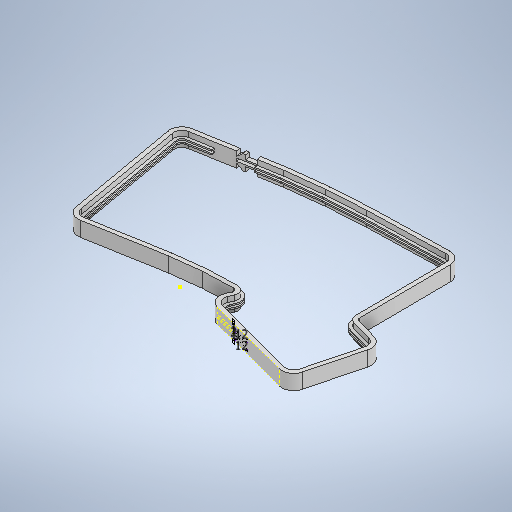
# Autodesk Inventor part: Case2.0_whole
Saved by Autodesk Inventor 2025 (Build 290162000, 162)
## iProperties
Created: 2024-07-14
Part Number: Case2.0_whole
Material: Generic
Document SubType Name: Modeling
Designer: ethan
Density: 1 g/cm^3
Appearance: Default
Author: ethan
Autodesk Inventor part; units mm, degrees
ref_plane "YZ Plane" through (0, 0, 0) normal (1, 0, 0) x (0, 1, 0)
ref_plane "XZ Plane" through (0, 0, 0) normal (0, 1, 0) x (-1, 0, 0)
sketch "Sketch1" plane through (0, 0, 0) normal (0, 1, 0) x (-1, 0, 0)
  line L0 (-82.0743, -49.0378) -> (-95.2699, 25.7981) construction
  line L1 (-91.2026, 31.5924) -> (-36.7795, 41.0576) construction
  line L2 (-36.5045, 41.0976) -> (-11.557, 44.02) construction
  line L3 (-11.2903, 44.0441) -> (14.1113, 45.648) construction
  line L4 (14.295, 45.6562) -> (66.1055, 47.0175) construction
  line L5 (71.2366, 42.0628) -> (71.7707, -19.1365) construction
  line L6 (75.3629, -23.8906) -> (89.6926, -28.0947) construction
  line L7 (93.1258, -34.1444) -> (84.0794, -69.1243) construction
  line L8 (77.9595, -72.706) -> (21.637, -57.8008) construction
  line L9 (18.302, -51.0413) -> (19.5764, -47.9879) construction
  line L10 (14.7916, -41.0649) -> (-5.2075, -41.7475) construction
  line L11 (-5.6408, -41.7811) -> (-26.0301, -44.2616) construction
  line L12 (-26.2924, -44.3006) -> (-76.2841, -53.0939) construction
  arc A0 (-91.2026, 31.5924) -> (-95.2699, 25.7981) centre (-90.3459, 26.6664) ccw construction
  arc A1 (-36.5045, 41.0976) -> (-36.7795, 41.0576) centre (-35.9227, 36.1315) ccw construction
  arc A2 (-11.2903, 44.0441) -> (-11.557, 44.02) centre (-10.9752, 39.054) ccw construction
  arc A3 (14.295, 45.6562) -> (14.1113, 45.648) centre (14.4264, 40.6579) ccw construction
  arc A4 (71.2366, 42.0628) -> (66.1055, 47.0175) centre (66.2368, 42.0192) ccw construction
  arc A5 (71.7707, -19.1365) -> (75.3629, -23.8906) centre (76.7705, -19.0928) ccw construction
  arc A6 (93.1258, -34.1444) -> (89.6926, -28.0947) centre (88.285, -32.8925) ccw construction
  arc A7 (77.9595, -72.706) -> (84.0794, -69.1243) centre (79.2386, -67.8724) ccw construction
  arc A8 (18.302, -51.0413) -> (21.637, -57.8008) centre (22.9162, -52.9672) ccw construction
  arc A9 (19.5764, -47.9879) -> (14.7916, -41.0649) centre (14.9621, -46.062) ccw construction
  arc A10 (-5.2075, -41.7475) -> (-5.6408, -41.7811) centre (-5.037, -46.7446) ccw construction
  arc A11 (-26.0301, -44.2616) -> (-26.2924, -44.3006) centre (-25.4262, -49.225) ccw construction
  arc A12 (-82.0743, -49.0378) -> (-76.2841, -53.0939) centre (-77.1503, -48.1695) ccw construction
  arc A13 (-91.2369, 31.7895) -> (-95.4669, 25.7634) centre (-90.3459, 26.6664) ccw
  line L13 (-91.2369, 31.7895) -> (-36.8137, 41.2546)
  arc A14 (-36.5277, 41.2962) -> (-36.8137, 41.2546) centre (-35.9227, 36.1315) ccw
  line L14 (-36.5277, 41.2962) -> (-11.5803, 44.2187)
  line L15 (-11.3029, 44.2437) -> (14.0987, 45.8476)
  arc A15 (-11.3029, 44.2437) -> (-11.5803, 44.2187) centre (-10.9752, 39.054) ccw
  arc A16 (14.2898, 45.8561) -> (14.0987, 45.8476) centre (14.4264, 40.6579) ccw
  line L16 (14.2898, 45.8561) -> (66.1002, 47.2174)
  arc A17 (71.4366, 42.0646) -> (66.1002, 47.2174) centre (66.2368, 42.0192) ccw
  line L17 (71.4366, 42.0646) -> (71.9707, -19.1347)
  arc A18 (71.9707, -19.1347) -> (75.4192, -23.6987) centre (76.7705, -19.0928) ccw
  line L18 (75.4192, -23.6987) -> (89.7489, -27.9028)
  arc A19 (93.3194, -34.1945) -> (89.7489, -27.9028) centre (88.285, -32.8925) ccw
  line L19 (93.3194, -34.1945) -> (84.273, -69.1743)
  arc A20 (77.9083, -72.8993) -> (84.273, -69.1743) centre (79.2386, -67.8724) ccw
  line L20 (77.9083, -72.8993) -> (21.5859, -57.9941)
  arc A21 (18.1174, -50.9643) -> (21.5859, -57.9941) centre (22.9162, -52.9672) ccw
  line L21 (18.1174, -50.9643) -> (19.3918, -47.9108)
  arc A22 (19.3918, -47.9108) -> (14.7984, -41.2648) centre (14.9621, -46.062) ccw
  line L22 (14.7984, -41.2648) -> (-5.2007, -41.9473)
  arc A23 (-5.2007, -41.9473) -> (-5.6167, -41.9797) centre (-5.037, -46.7446) ccw
  line L23 (-5.6167, -41.9797) -> (-26.0059, -44.4601)
  arc A24 (-26.0059, -44.4601) -> (-26.2578, -44.4975) centre (-25.4262, -49.225) ccw
  line L24 (-26.2578, -44.4975) -> (-76.2494, -53.2909)
  arc A25 (-82.2713, -49.0725) -> (-76.2494, -53.2909) centre (-77.1503, -48.1695) ccw
  line L25 (-82.2713, -49.0725) -> (-95.4669, 25.7634)
  arc A26 (-91.7166, 34.5481) -> (-98.2243, 25.2772) centre (-90.3459, 26.6664) ccw
  line L26 (-91.7166, 34.5481) -> (-37.2935, 44.0132)
  line L27 (-36.8535, 44.0772) -> (-11.906, 46.9997)
  arc A27 (-36.8535, 44.0772) -> (-37.2935, 44.0132) centre (-35.9227, 36.1315) ccw
  arc A28 (-11.4794, 47.0381) -> (-11.906, 46.9997) centre (-10.9752, 39.054) ccw
  line L28 (-11.4794, 47.0381) -> (13.9222, 48.642)
  arc A29 (14.2162, 48.6551) -> (13.9222, 48.642) centre (14.4264, 40.6579) ccw
  line L29 (14.2162, 48.6551) -> (66.0267, 50.0164)
  arc A30 (74.2365, 42.089) -> (66.0267, 50.0164) centre (66.2368, 42.0192) ccw
  line L30 (74.2365, 42.089) -> (74.7706, -19.1103)
  arc A31 (74.7706, -19.1103) -> (76.2074, -21.0119) centre (76.7705, -19.0928) ccw
  line L31 (76.2074, -21.0119) -> (90.5372, -25.2161)
  arc A32 (96.0302, -34.8956) -> (90.5372, -25.2161) centre (88.285, -32.8925) ccw
  line L32 (96.0302, -34.8956) -> (86.9838, -69.8754)
  arc A33 (77.192, -75.6061) -> (86.9838, -69.8754) centre (79.2386, -67.8724) ccw
  line L33 (77.192, -75.6061) -> (20.8695, -60.7009)
  arc A34 (15.5334, -49.8859) -> (20.8695, -60.7009) centre (22.9162, -52.9672) ccw
  arc A35 (16.8078, -46.8324) -> (14.8939, -44.0632) centre (14.9621, -46.062) ccw
  line L34 (15.5334, -49.8859) -> (16.8078, -46.8324)
  line L35 (14.8939, -44.0632) -> (-5.1052, -44.7457)
  arc A36 (-5.1052, -44.7457) -> (-5.2785, -44.7592) centre (-5.037, -46.7446) ccw
  line L36 (-5.2785, -44.7592) -> (-25.6678, -47.2396)
  arc A37 (-25.6678, -47.2396) -> (-25.7727, -47.2552) centre (-25.4262, -49.225) ccw
  line L37 (-25.7727, -47.2552) -> (-75.7644, -56.0486)
  line L38 (-85.0287, -49.5587) -> (-98.2243, 25.2772)
  arc A38 (-85.0287, -49.5587) -> (-75.7644, -56.0486) centre (-77.1503, -48.1695) ccw
  point P0 (-26.1615, -44.2793)
  point P1 (-5.4246, -41.7596)
  point P2 (14.2031, 45.6529)
  point P3 (-25.7727, -47.2552)
  point P4 (-25.6678, -47.2396)
  point P5 (-5.2785, -44.7592)
  point P6 (-5.1052, -44.7457)
  point P7 (14.8939, -44.0632)
  point P8 (16.8078, -46.8324)
  point P9 (76.2074, -21.0119)
  point P10 (74.7706, -19.1103)
  point P11 (74.2365, 42.089)
  point P12 (-11.5803, 44.2187)
  point P13 (71.9707, -19.1347)
  point P14 (75.4192, -23.6987)
  point P15 (-5.2007, -41.9473)
  point P16 (-5.6167, -41.9797)
  point P17 (-26.2578, -44.4975)
  point P18 (-95.4669, 25.7634)
  dimension "d8" = 0.2
  dimension "d9" = 0.2
  dimension "d10" = 0.2
  dimension "d11" = 0.2
  dimension "d12" = 0.2
  dimension "d13" = 0.2
  dimension "d14" = 0.2
  dimension "d15" = 0.2
  dimension "d16" = 0.2
  dimension "d17" = 0.2
  dimension "d18" = 0.2
  dimension "d19" = 0.2
  dimension "d20" = 0.2
  dimension "d21" = 0.2
  dimension "d22" = 0.2
  dimension "d23" = 0.2
  dimension "d24" = 0.2
  dimension "d25" = 0.2
  dimension "d26" = 0.2
  dimension "d27" = 0.2
  dimension "d28" = 0.2
  dimension "d29" = 0.2
  dimension "d30" = 0.2
  dimension "d31" = 0.2
  dimension "d32" = 0.2
  dimension "d33" = 0.2
  dimension "d34" = 2.8
  dimension "d35" = 2.8
  dimension "d36" = 2.8
  dimension "d37" = 2.8
  dimension "d38" = 2.8
  dimension "d39" = 2.8
  dimension "d40" = 2.8
  dimension "d41" = 2.8
  dimension "d42" = 2.8
  dimension "d43" = 2.8
  dimension "d44" = 2.8
  dimension "d45" = 2.8
  dimension "d46" = 2.8
  dimension "d47" = 2.8
  dimension "d48" = 2.8
  dimension "d49" = 2.8
  dimension "d50" = 2.8
  dimension "d51" = 2.8
  dimension "d52" = 2.8
  dimension "d53" = 2.8
  dimension "d54" = 2.8
  dimension "d55" = 2.8
  dimension "d56" = 2.8
  dimension "d57" = 2.8
  dimension "d58" = 2.8
  dimension "d59" = 2.8
  constraints: 81 point on circle, 78 end point, 39 centre point, 26 parallel, 33 other
  measures "d8" radial gap between concentric circles of A0 A13
  measures "d9" distance between parallel lines of L1 L13
  measures "d10" radial gap between concentric circles of A1 A14
  measures "d11" distance between parallel lines of L2 L14
  measures "d12" distance between parallel lines of L3 L15
  measures "d13" radial gap between concentric circles of A2 A15
  measures "d14" radial gap between concentric circles of A3 A16
  measures "d15" distance between parallel lines of L4 L16
  measures "d16" radial gap between concentric circles of A4 A17
  measures "d17" distance between parallel lines of L5 L17
  measures "d18" radial gap between concentric circles of A5 A18
  measures "d19" distance between parallel lines of L6 L18
  measures "d20" radial gap between concentric circles of A6 A19
  measures "d21" distance between parallel lines of L7 L19
  measures "d22" radial gap between concentric circles of A7 A20
  measures "d23" distance between parallel lines of L8 L20
  measures "d24" radial gap between concentric circles of A8 A21
  measures "d25" distance between parallel lines of L9 L21
  measures "d26" radial gap between concentric circles of A9 A22
  measures "d27" distance between parallel lines of L10 L22
  measures "d28" radial gap between concentric circles of A10 A23
  measures "d29" distance between parallel lines of L11 L23
  measures "d30" radial gap between concentric circles of A11 A24
  measures "d31" distance between parallel lines of L12 L24
  measures "d32" radial gap between concentric circles of A12 A25
  measures "d33" distance between parallel lines of L0 L25
  measures "d34" radial gap between concentric circles of A13 A26
  measures "d35" distance between parallel lines of L13 L26
  measures "d36" distance between parallel lines of L14 L27
  measures "d37" radial gap between concentric circles of A14 A27
  measures "d38" radial gap between concentric circles of A15 A28
  measures "d39" distance between parallel lines of L15 L28
  measures "d40" radial gap between concentric circles of A16 A29
  measures "d41" distance between parallel lines of L16 L29
  measures "d42" radial gap between concentric circles of A17 A30
  measures "d43" distance between parallel lines of L17 L30
  measures "d44" radial gap between concentric circles of A18 A31
  measures "d45" distance between parallel lines of L18 L31
  measures "d46" radial gap between concentric circles of A19 A32
  measures "d47" distance between parallel lines of L19 L32
  measures "d48" radial gap between concentric circles of A20 A33
  measures "d49" distance between parallel lines of L20 L33
  measures "d50" radial gap between concentric circles of A21 A34
  measures "d51" radial gap between concentric circles of A22 A35
  measures "d52" distance between parallel lines of L21 L34
  measures "d53" distance between parallel lines of L22 L35
  measures "d54" radial gap between concentric circles of A23 A36
  measures "d55" distance between parallel lines of L23 L36
  measures "d56" radial gap between concentric circles of A24 A37
  measures "d57" distance between parallel lines of L24 L37
  measures "d58" distance between parallel lines of L25 L38
  measures "d59" radial gap between concentric circles of A25 A38
extrude "Body" add sketch "Sketch1" along normal blind 10
ref_plane "Midplane" through (0, 5, 0) normal (0, 1, 0) x (1, 0, 0)
sketch "Sketch2" plane through (0, 5, 0) normal (0, 1, 0) x (1, 0, 0)
  line L0 (37.2935, -44.0132) -> (91.7166, -34.5481) projected
  arc A0 (91.7166, -34.5481) -> (98.2243, -25.2772) centre (90.3459, -26.6664) ccw projected
  line L1 (98.2243, -25.2772) -> (85.0287, 49.5587) projected
  arc A1 (85.0287, 49.5587) -> (75.7644, 56.0486) centre (77.1503, 48.1695) ccw projected
  line L2 (75.7644, 56.0486) -> (25.7727, 47.2552) projected
  arc A2 (25.6678, 47.2396) -> (25.7727, 47.2552) centre (25.4262, 49.225) ccw projected
  line L3 (25.6678, 47.2396) -> (5.2785, 44.7592) projected
  arc A3 (5.1052, 44.7457) -> (5.2785, 44.7592) centre (5.037, 46.7446) ccw projected
  line L4 (5.1052, 44.7457) -> (-14.8939, 44.0632) projected
  arc A4 (-16.8078, 46.8324) -> (-14.8939, 44.0632) centre (-14.9621, 46.062) ccw projected
  line L5 (-16.8078, 46.8324) -> (-15.5334, 49.8859) projected
  arc A5 (-15.5334, 49.8859) -> (-20.8695, 60.7009) centre (-22.9162, 52.9672) ccw projected
  line L6 (-20.8695, 60.7009) -> (-77.192, 75.6061) projected
  arc A6 (-77.192, 75.6061) -> (-86.9838, 69.8754) centre (-79.2386, 67.8724) ccw projected
  line L7 (-86.9838, 69.8754) -> (-96.0302, 34.8956) projected
  arc A7 (-96.0302, 34.8956) -> (-90.5372, 25.2161) centre (-88.285, 32.8925) ccw projected
  line L8 (-90.5372, 25.2161) -> (-76.2074, 21.0119) projected
  arc A8 (-74.7706, 19.1103) -> (-76.2074, 21.0119) centre (-76.7705, 19.0928) ccw projected
  line L9 (-74.7706, 19.1103) -> (-74.2365, -42.089) projected
  arc A9 (-74.2365, -42.089) -> (-66.0267, -50.0164) centre (-66.2368, -42.0192) ccw projected
  line L10 (-66.0267, -50.0164) -> (-14.2162, -48.6551) projected
  arc A10 (-14.2162, -48.6551) -> (-13.9222, -48.642) centre (-14.4264, -40.6579) ccw projected
  line L11 (-13.9222, -48.642) -> (11.4794, -47.0381) projected
  arc A11 (11.4794, -47.0381) -> (11.906, -46.9997) centre (10.9752, -39.054) ccw projected
  line L12 (11.906, -46.9997) -> (36.8535, -44.0772) projected
  arc A12 (36.8535, -44.0772) -> (37.2935, -44.0132) centre (35.9227, -36.1315) ccw projected
  line L13 (36.5277, -41.2962) -> (11.5803, -44.2187) projected
  arc A13 (11.3029, -44.2437) -> (11.5803, -44.2187) centre (10.9752, -39.054) ccw projected
  line L14 (11.3029, -44.2437) -> (-14.0987, -45.8476) projected
  arc A14 (-14.2898, -45.8561) -> (-14.0987, -45.8476) centre (-14.4264, -40.6579) ccw projected
  line L15 (-14.2898, -45.8561) -> (-66.1002, -47.2174) projected
  arc A15 (-71.4366, -42.0646) -> (-66.1002, -47.2174) centre (-66.2368, -42.0192) ccw projected
  line L16 (-71.4366, -42.0646) -> (-71.9707, 19.1347) projected
  arc A16 (-71.9707, 19.1347) -> (-75.4192, 23.6987) centre (-76.7705, 19.0928) ccw projected
  line L17 (-75.4192, 23.6987) -> (-89.7489, 27.9028) projected
  arc A17 (-93.3194, 34.1945) -> (-89.7489, 27.9028) centre (-88.285, 32.8925) ccw projected
  line L18 (-93.3194, 34.1945) -> (-84.273, 69.1743) projected
  arc A18 (-77.9083, 72.8993) -> (-84.273, 69.1743) centre (-79.2386, 67.8724) ccw projected
  line L19 (-77.9083, 72.8993) -> (-21.5859, 57.9941) projected
  arc A19 (-18.1174, 50.9643) -> (-21.5859, 57.9941) centre (-22.9162, 52.9672) ccw projected
  line L20 (-18.1174, 50.9643) -> (-19.3918, 47.9108) projected
  arc A20 (-19.3918, 47.9108) -> (-14.7984, 41.2648) centre (-14.9621, 46.062) ccw projected
  line L21 (-14.7984, 41.2648) -> (5.2007, 41.9473) projected
  arc A21 (5.2007, 41.9473) -> (5.6167, 41.9797) centre (5.037, 46.7446) ccw projected
  line L22 (5.6167, 41.9797) -> (26.0059, 44.4601) projected
  arc A22 (26.0059, 44.4601) -> (26.2578, 44.4975) centre (25.4262, 49.225) ccw projected
  line L23 (26.2578, 44.4975) -> (76.2494, 53.2909) projected
  arc A23 (82.2713, 49.0725) -> (76.2494, 53.2909) centre (77.1503, 48.1695) ccw projected
  line L24 (82.2713, 49.0725) -> (95.4669, -25.7634) projected
  arc A24 (91.2369, -31.7895) -> (95.4669, -25.7634) centre (90.3459, -26.6664) ccw projected
  line L25 (91.2369, -31.7895) -> (36.8137, -41.2546) projected
  arc A25 (36.5277, -41.2962) -> (36.8137, -41.2546) centre (35.9227, -36.1315) ccw projected
  line L26 (-82.3367, 68.6736) -> (-91.3831, 33.6937)
  arc A26 (-91.3831, 33.6937) -> (-89.1859, 29.8219) centre (-88.285, 32.8925) ccw
  line L27 (-89.1859, 29.8219) -> (-74.8562, 25.6178)
  arc A27 (-69.9707, 19.1522) -> (-74.8562, 25.6178) centre (-76.7705, 19.0928) ccw
  line L28 (-69.9707, 19.1522) -> (-69.4367, -42.0471)
  arc A28 (-69.4367, -42.0471) -> (-66.1527, -45.2181) centre (-66.2368, -42.0192) ccw
  line L29 (-66.1527, -45.2181) -> (-14.3423, -43.8568)
  arc A29 (-14.3423, -43.8568) -> (-14.2247, -43.8515) centre (-14.4264, -40.6579) ccw
  line L30 (-14.2247, -43.8515) -> (11.1769, -42.2476)
  arc A30 (11.1769, -42.2476) -> (11.3476, -42.2323) centre (10.9752, -39.054) ccw
  line L31 (11.3476, -42.2323) -> (36.295, -39.3098)
  arc A31 (36.295, -39.3098) -> (36.471, -39.2842) centre (35.9227, -36.1315) ccw
  line L32 (36.471, -39.2842) -> (90.8942, -29.819)
  arc A32 (90.8942, -29.819) -> (93.4972, -26.1107) centre (90.3459, -26.6664) ccw
  line L33 (93.4972, -26.1107) -> (80.3017, 48.7252)
  arc A33 (80.3017, 48.7252) -> (76.5959, 51.3212) centre (77.1503, 48.1695) ccw
  line L34 (76.5959, 51.3212) -> (26.6043, 42.5278)
  arc A34 (26.2474, 42.4747) -> (26.6043, 42.5278) centre (25.4262, 49.225) ccw
  line L35 (26.2474, 42.4747) -> (5.8582, 39.9943)
  arc A35 (5.2689, 39.9485) -> (5.8582, 39.9943) centre (5.037, 46.7446) ccw
  line L36 (5.2689, 39.9485) -> (-14.7302, 39.266)
  arc A36 (-21.2375, 48.6811) -> (-14.7302, 39.266) centre (-14.9621, 46.062) ccw
  line L37 (-21.2375, 48.6811) -> (-19.9631, 51.7346)
  arc A37 (-19.9631, 51.7346) -> (-22.0975, 56.0607) centre (-22.9162, 52.9672) ccw
  line L38 (-22.0975, 56.0607) -> (-78.42, 70.9659)
  arc A38 (-78.42, 70.9659) -> (-82.3367, 68.6736) centre (-79.2386, 67.8724) ccw
  line L39 (63.6826, -34.5516) -> (64.0253, -36.522)
  line L40 (75.9977, -32.4098) -> (76.3404, -34.3802)
  line L41 (76.3404, -34.3802) -> (51.7102, -38.6639)
  line L42 (51.7102, -38.6639) -> (51.3675, -36.6934)
  line L43 (51.3675, -36.6934) -> (75.9977, -32.4098)
  line L44 (75.9977, -32.4098) -> (51.7102, -38.6639) construction
  line L45 (76.3404, -34.3802) -> (51.3675, -36.6934) construction
  line L46 (-50.2588, 63.5133) -> (-49.7471, 65.4467)
  line L47 (-61.8311, 68.6446) -> (-62.3428, 66.7112)
  line L48 (-62.3428, 66.7112) -> (-38.1747, 60.3154)
  line L49 (-38.1747, 60.3154) -> (-37.6631, 62.2488)
  line L50 (-37.6631, 62.2488) -> (-61.8311, 68.6446)
  line L51 (-61.8311, 68.6446) -> (-38.1747, 60.3154) construction
  line L52 (-62.3428, 66.7112) -> (-37.6631, 62.2488) construction
  point P0 (0, 0)
  point P1 (63.8539, -35.5368)
  point P2 (51.7102, -38.6639)
  point P3 (51.3675, -36.6934)
  point P4 (75.9977, -32.4098)
  point P5 (76.3404, -34.3802)
  point P6 (-50.0029, 64.48)
  point P7 (-61.8311, 68.6446)
  point P8 (-38.1747, 60.3154)
  dimension "d62" = 2
  dimension "d67" = 25
  dimension "d68" = 25
  constraints: 54 end point, 26 point on circle, 13 centre point, 10 midpoint, 5 parallel, 3 perpendicular, 25 other
  measures "d62" distance between parallel lines of L18 L26
  measures "d67" distance of L40.end L41.end
  measures "d68" distance of L48.end L47.end
extrude "Groove-Outer" add sketch "Sketch2" along normal mid plane 3 contours L13 A13 L14 A14 L15 A15 L16 A16 L17 A17 L18 A18 L19 L47 L38 A38 L26 A26 L27 A27 L28 A28 L29 A29 L30 A30 L31 A31 L32 L42 L25 A25 | L40 L32 A32 L33 A33 L34 A34 L35 A35 L36 A36 L37 A37 L38 L49 L19 A19 L20 A20 L21 A21 L22 A22 L23 A23 L24 A24 L25
sketch "Sketch3" plane through (0, 5, 0) normal (0, 1, 0) x (1, 0, 0)
  line L0 (82.2713, 49.0725) -> (95.4669, -25.7634) projected
  arc A0 (82.2713, 49.0725) -> (76.2494, 53.2909) centre (77.1503, 48.1695) ccw projected
  line L1 (26.2578, 44.4975) -> (76.2494, 53.2909) projected
  arc A1 (26.0059, 44.4601) -> (26.2578, 44.4975) centre (25.4262, 49.225) ccw projected
  line L2 (5.6167, 41.9797) -> (26.0059, 44.4601) projected
  arc A2 (5.2007, 41.9473) -> (5.6167, 41.9797) centre (5.037, 46.7446) ccw projected
  line L3 (-14.7984, 41.2648) -> (5.2007, 41.9473) projected
  arc A3 (-19.3918, 47.9108) -> (-14.7984, 41.2648) centre (-14.9621, 46.062) ccw projected
  line L4 (-18.1174, 50.9643) -> (-19.3918, 47.9108) projected
  arc A4 (-18.1174, 50.9643) -> (-21.5859, 57.9941) centre (-22.9162, 52.9672) ccw projected
  line L5 (-77.9083, 72.8993) -> (-61.8311, 68.6446) projected
  arc A5 (-77.9083, 72.8993) -> (-84.273, 69.1743) centre (-79.2386, 67.8724) ccw projected
  line L6 (-93.3194, 34.1945) -> (-84.273, 69.1743) projected
  arc A6 (-93.3194, 34.1945) -> (-89.7489, 27.9028) centre (-88.285, 32.8925) ccw projected
  line L7 (-75.4192, 23.6987) -> (-89.7489, 27.9028) projected
  arc A7 (-71.9707, 19.1347) -> (-75.4192, 23.6987) centre (-76.7705, 19.0928) ccw projected
  line L8 (-71.4366, -42.0646) -> (-71.9707, 19.1347) projected
  arc A8 (-71.4366, -42.0646) -> (-66.1002, -47.2174) centre (-66.2368, -42.0192) ccw projected
  line L9 (-14.2898, -45.8561) -> (-66.1002, -47.2174) projected
  arc A9 (-14.2898, -45.8561) -> (-14.0987, -45.8476) centre (-14.4264, -40.6579) ccw projected
  line L10 (11.3029, -44.2437) -> (-14.0987, -45.8476) projected
  arc A10 (11.3029, -44.2437) -> (11.5803, -44.2187) centre (10.9752, -39.054) ccw projected
  line L11 (36.5277, -41.2962) -> (11.5803, -44.2187) projected
  arc A11 (36.5277, -41.2962) -> (36.8137, -41.2546) centre (35.9227, -36.1315) ccw projected
  line L12 (51.7102, -38.6639) -> (36.8137, -41.2546) projected
  arc A12 (91.2369, -31.7895) -> (95.4669, -25.7634) centre (90.3459, -26.6664) ccw projected
  arc A13 (-21.2375, 48.6811) -> (-14.7302, 39.266) centre (-14.9621, 46.062) ccw projected
  line L13 (-14.7302, 39.266) -> (5.2689, 39.9485) projected
  arc A14 (5.2689, 39.9485) -> (5.8582, 39.9943) centre (5.037, 46.7446) ccw projected
  line L14 (5.8582, 39.9943) -> (26.2474, 42.4747) projected
  arc A15 (26.2474, 42.4747) -> (26.6043, 42.5278) centre (25.4262, 49.225) ccw projected
  line L15 (26.6043, 42.5278) -> (76.5959, 51.3212) projected
  arc A16 (80.3017, 48.7252) -> (76.5959, 51.3212) centre (77.1503, 48.1695) ccw projected
  line L16 (80.3017, 48.7252) -> (93.4972, -26.1107) projected
  arc A17 (90.8942, -29.819) -> (93.4972, -26.1107) centre (90.3459, -26.6664) ccw projected
  line L17 (90.8942, -29.819) -> (75.9977, -32.4098) projected
  arc A18 (36.295, -39.3098) -> (36.471, -39.2842) centre (35.9227, -36.1315) ccw projected
  line L18 (36.295, -39.3098) -> (11.3476, -42.2323) projected
  arc A19 (11.1769, -42.2476) -> (11.3476, -42.2323) centre (10.9752, -39.054) ccw projected
  line L19 (11.1769, -42.2476) -> (-14.2247, -43.8515) projected
  arc A20 (-14.3423, -43.8568) -> (-14.2247, -43.8515) centre (-14.4264, -40.6579) ccw projected
  line L20 (-14.3423, -43.8568) -> (-66.1527, -45.2181) projected
  arc A21 (-69.4367, -42.0471) -> (-66.1527, -45.2181) centre (-66.2368, -42.0192) ccw projected
  line L21 (-69.4367, -42.0471) -> (-69.9707, 19.1522) projected
  arc A22 (-69.9707, 19.1522) -> (-74.8562, 25.6178) centre (-76.7705, 19.0928) ccw projected
  line L22 (-74.8562, 25.6178) -> (-89.1859, 29.8219) projected
  arc A23 (-91.3831, 33.6937) -> (-89.1859, 29.8219) centre (-88.285, 32.8925) ccw projected
  line L23 (-91.3831, 33.6937) -> (-82.3367, 68.6736) projected
  arc A24 (-78.42, 70.9659) -> (-82.3367, 68.6736) centre (-79.2386, 67.8724) ccw projected
  line L24 (-78.42, 70.9659) -> (-62.3428, 66.7112) projected
  arc A25 (-19.9631, 51.7346) -> (-22.0975, 56.0607) centre (-22.9162, 52.9672) ccw projected
  line L25 (-19.9631, 51.7346) -> (-21.2375, 48.6811) projected
  line L26 (51.7102, -38.6639) -> (51.3675, -36.6934) projected
  line L27 (51.3675, -36.6934) -> (36.471, -39.2842) projected
  line L28 (75.9977, -32.4098) -> (76.3404, -34.3802) projected
  line L29 (91.2369, -31.7895) -> (76.3404, -34.3802) projected
  line L30 (-62.3428, 66.7112) -> (-61.8311, 68.6446) projected
  line L31 (-37.6631, 62.2488) -> (-21.5859, 57.9941) projected
  line L32 (-37.6631, 62.2488) -> (-38.1747, 60.3154) projected
  line L33 (-38.1747, 60.3154) -> (-22.0975, 56.0607) projected
  point P0 (0, 0)
extrude "Groove" cut sketch "Sketch3" along normal mid plane 1.2
sketch "Sketch4" plane through (91.7166, 0, 34.5481) normal (0.1713, 0, 0.9852) x (0.9852, 0, -0.1713)
  line L0 (-55.2401, 0) -> (0, 0) construction
  line L1 (0, 0) -> (0, 10) construction
  line L2 (-55.2401, 10) -> (0, 10) construction
  line L3 (-55.2401, 0) -> (-55.2401, 10) construction
  line L4 (-40.12, 5.6) -> (-55.2401, 5.6) construction
  line L5 (-55.2401, 5.6) -> (-55.2401, 6.5) construction
  line L6 (-40.12, 6.5) -> (-55.2401, 6.5) construction
  line L7 (-40.12, 5.6) -> (-40.12, 6.5) construction
  line L8 (-55.2401, 4.4) -> (-40.12, 4.4) construction
  line L9 (-40.12, 3.5) -> (-40.12, 4.4) construction
  line L10 (-55.2401, 3.5) -> (-40.12, 3.5) construction
  line L11 (-55.2401, 3.5) -> (-55.2401, 4.4) construction
  line L12 (0, 5.6) -> (-15.12, 5.6) construction
  line L13 (-15.12, 5.6) -> (-15.12, 6.5) construction
  line L14 (0, 6.5) -> (-15.12, 6.5) construction
  line L15 (0, 5.6) -> (0, 6.5) construction
  line L16 (-15.12, 4.4) -> (0, 4.4) construction
  line L17 (0, 3.5) -> (0, 4.4) construction
  line L18 (-15.12, 3.5) -> (0, 3.5) construction
  line L19 (-15.12, 3.5) -> (-15.12, 4.4) construction
  line L20 (-40.12, 0) -> (-40.12, 10) construction
  line L21 (-15.12, 0) -> (-15.12, 10) construction
  line L22 (-40.12, 5) -> (-40.12, 6) construction
  line L23 (-40.12, 6) -> (-40.12, 4) construction
  line L24 (-40.12, 6) -> (-40.12, 7) construction
  line L25 (-40.12, 7) -> (-33.3521, 7) construction
  line L26 (-28.12, 7) -> (-28.12, 6) construction
  line L27 (-28.12, 6) -> (-40.12, 6) construction
  line L28 (-40.12, 4) -> (-40.12, 3) construction
  line L29 (-40.12, 3) -> (-33.3521, 3) construction
  line L30 (-28.12, 3) -> (-28.12, 4) construction
  line L31 (-28.12, 4) -> (-40.12, 4) construction
  line L32 (-28.12, 3) -> (-31.8521, 0) construction
  line L33 (-31.8521, 0) -> (-33.3521, 0) construction
  line L34 (-33.3521, 0) -> (-33.3521, 3) construction
  line L35 (-28.12, 7) -> (-31.8521, 10) construction
  line L36 (-31.8521, 10) -> (-33.3521, 10) construction
  line L37 (-33.3521, 10) -> (-33.3521, 7) construction
  line L38 (-40.12, 7) -> (-33.3521, 7)
  line L39 (-33.3521, 7) -> (-33.3521, 10)
  line L40 (-33.3521, 10) -> (-31.8521, 10)
  line L41 (-55.2401, 10) -> (0, 10) projected
  line L42 (-28.12, 7) -> (-31.8521, 10)
  line L43 (-28.12, 6) -> (-28.12, 7)
  line L44 (-28.12, 6) -> (-40.12, 6)
  line L45 (-40.12, 7) -> (-40.12, 10)
  line L46 (-40.12, 10) -> (-33.3521, 10)
  line L47 (-40.12, 3) -> (-33.3521, 3)
  line L48 (-33.3521, 3) -> (-33.3521, 0)
  line L49 (-33.3521, 0) -> (-40.12, 0)
  line L50 (-40.12, 0) -> (-40.12, 3)
  line L51 (-40.12, 4) -> (-28.12, 4)
  line L52 (-28.12, 4) -> (-28.12, 6)
  line L53 (-28.12, 6) -> (-40.12, 6)
  line L54 (-40.12, 6) -> (-40.12, 4)
  line L55 (-28.12, 3) -> (-28.12, 0)
  line L56 (-31.8521, 0) -> (-28.12, 0)
  line L57 (-31.8521, 0) -> (-28.12, 3)
  line L58 (-40.12, 10) -> (-33.3521, 10)
  line L59 (-33.3521, 10) -> (-33.3521, 7)
  line L60 (-33.3521, 7) -> (-40.12, 7)
  line L61 (-40.12, 7) -> (-40.12, 10)
  line L62 (-28.12, 7) -> (-28.12, 10)
  line L63 (-28.12, 10) -> (-31.8521, 10)
  point P0 (-84.4406, 0)
  point P1 (-40.12, 6)
  dimension "d69" = 1
  dimension "d70" = 2
  dimension "d71" = 1
  dimension "d72" = 12
  dimension "d73" = 1
  dimension "d74" = 12
  dimension "d76" = 1.5
  dimension "d77" = 1.5
  constraints: 86 end point, 16 perpendicular, 14 point on line, 10 parallel, 5 collinear, 3 horizontal, 1 midpoint
  measures "d69" distance of L22.start L22.end
  measures "d70" distance of L22.end L23.end
  measures "d71" distance of L22.end L24.end
  measures "d72" distance of L24.end L26.start
  measures "d73" distance of L23.end L28.end
  measures "d74" distance of L30.start L28.end
  measures "d76" distance of L32.end L33.end
  measures "d77" distance of L35.end L36.end
extrude "Extrusion4" cut sketch "Sketch4" against normal blind 10
sketch "Sketch5" plane through (-77.192, 0, -75.6061) normal (0.2558, 0, -0.9667) x (-0.9667, 0, -0.2558)
  line L0 (-58.2613, 0) -> (0, 0) construction
  line L1 (0, 0) -> (0, 10) construction
  line L2 (-58.2613, 10) -> (0, 10) construction
  line L3 (-58.2613, 0) -> (-58.2613, 10) construction
  line L4 (-58.2613, 3.5) -> (-41.6307, 3.5) construction
  line L5 (-41.6307, 4.4) -> (-58.2613, 4.4) construction
  line L6 (-58.2613, 5.6) -> (-41.6307, 5.6) construction
  line L7 (-41.6307, 6.5) -> (-58.2613, 6.5) construction
  line L8 (-41.6307, 0) -> (-41.6307, 10) construction
  line L9 (-41.6307, 5) -> (-41.6307, 6) construction
  line L10 (-41.6307, 6) -> (-41.6307, 4) construction
  line L11 (-41.6307, 6) -> (-41.6307, 7) construction
  line L12 (-41.6307, 7) -> (-29.6307, 7) construction
  line L13 (-29.6307, 7) -> (-29.6307, 6) construction
  line L14 (-29.6307, 6) -> (-41.6307, 6) construction
  line L15 (-41.6307, 4) -> (-41.6307, 3) construction
  line L16 (-41.6307, 3) -> (-29.6307, 3) construction
  line L17 (-29.6307, 3) -> (-29.6307, 4) construction
  line L18 (-29.6307, 4) -> (-41.6307, 4) construction
  point P0 (-93.9657, 0)
  dimension "d80" = 1
  dimension "d81" = 2
  dimension "d82" = 1
  dimension "d83" = 12
  dimension "d84" = 1
  dimension "d85" = 12
  constraints: 22 end point, 6 point on line, 4 parallel, 3 perpendicular, 1 midpoint
  measures "d80" distance of L9.start L9.end
  measures "d81" distance of L9.end L10.end
  measures "d82" distance of L9.end L11.end
  measures "d83" distance of L11.end L12.end
  measures "d84" distance of L10.end L15.end
  measures "d85" distance of L16.end L15.end
body "Solid1"
